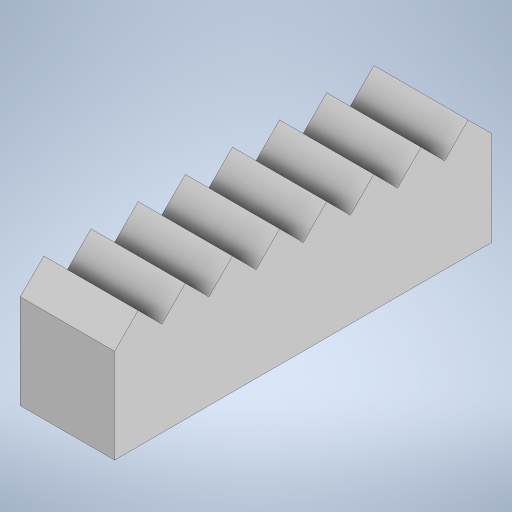
# Autodesk Inventor part: Finger Rack
Saved by Autodesk Inventor 2023 (Build 270158000, 158)
## iProperties
Created: 2023-09-27
Part Number: Finger Rack
Material: Generic
Document SubType Name: Modeling
Designer: Turnt
Density: 1 g/cm^3
Appearance: Default
Author: Turnt
Autodesk Inventor part; units mm, degrees
ref_plane "YZ Plane" through (0, 0, 0) normal (1, 0, 0) x (0, 1, 0)
ref_plane "XZ Plane" through (0, 0, 0) normal (0, 1, 0) x (-1, 0, 0)
ref_plane "XY Plane" through (0, 0, 0) normal (0, 0, 1) x (1, 0, 0)
sketch "Sketch1" plane through (0, 0, 0) normal (0, 0, 1) x (1, 0, 0)
  line L0 (0, 0) -> (12.7, 0)
  line L1 (12.7, 0) -> (12.7, 12.7)
  line L2 (12.7, 12.7) -> (0, 12.7)
  line L3 (0, 12.7) -> (0, 0)
  dimension "d0" = 12.7
  dimension "d1" = 12.7
  constraints: 8 end point, 2 parallel, 1 horizontal, 1 perpendicular
  measures "d0" distance of L2.end L1.end
  measures "d1" distance of L1.end L0.end
extrude "Extrusion1" add sketch "Sketch1" along normal blind 50.8
sketch "Sketch2" plane through (12.7, 0, 0) normal (1, 0, 0) x (0, 0, -1)
  line L0 (-50.8, 0) -> (-50.8, 12.7) projected
  line L1 (-50.8, 12.7) -> (-44.45, 12.7)
  line L2 (0, 12.7) -> (-50.8, 12.7) projected
  line L3 (-50.8, 12.7) -> (-47.625, 15.875)
  line L4 (-50.8, 12.7) -> (-46.3099, 12.7) construction
  line L5 (-47.625, 15.875) -> (-44.45, 12.7)
  line L6 (-44.45, 12.7) -> (-41.275, 15.875)
  line L7 (-41.275, 15.875) -> (-38.1, 12.7)
  line L8 (-44.45, 12.7) -> (-38.1, 12.7)
  line L9 (-38.1, 12.7) -> (-34.925, 15.875)
  line L10 (-34.925, 15.875) -> (-31.75, 12.7)
  line L11 (-38.1, 12.7) -> (-31.75, 12.7)
  line L12 (-31.75, 12.7) -> (-28.575, 15.875)
  line L13 (-28.575, 15.875) -> (-25.4, 12.7)
  line L14 (-31.75, 12.7) -> (-25.4, 12.7)
  line L15 (-25.4, 12.7) -> (-22.225, 15.875)
  line L16 (-22.225, 15.875) -> (-19.05, 12.7)
  line L17 (-25.4, 12.7) -> (-19.05, 12.7)
  line L18 (-19.05, 12.7) -> (-15.875, 15.875)
  line L19 (-15.875, 15.875) -> (-12.7, 12.7)
  line L20 (-19.05, 12.7) -> (-12.7, 12.7)
  line L21 (-12.7, 12.7) -> (-9.525, 15.875)
  line L22 (-9.525, 15.875) -> (-6.35, 12.7)
  line L23 (-12.7, 12.7) -> (-6.35, 12.7)
  line L24 (-6.35, 12.7) -> (-3.175, 15.875)
  line L25 (-3.175, 15.875) -> (0, 12.7)
  line L26 (-6.35, 12.7) -> (0, 12.7)
  line L27 (-47.625, 15.875) -> (-47.625, 12.7) construction
  point P0 (0, 0)
  dimension "d8" = 45
  dimension "d11" = 6.35
  dimension "d18" = 3.175
  constraints: 52 end point, 2 horizontal, 2 perpendicular, 2 point on line, 1 equal length, 42 other
  measures "d8" angle of L4 L3
  measures "d11" distance of L0.end L6.start
  measures "d18" distance of L3.end L27.end
extrude "Extrusion2" add sketch "Sketch2" against normal blind 12.7
body "Solid1"
